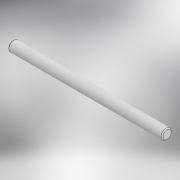
# Autodesk Inventor part: 绞杆
Saved by Autodesk Inventor 2020 (Build 240168000, 168)
## iProperties
Created: 2021-05-02
Part Number: 绞杆
Material: 常规
Document SubType Name: Modeling
Designer: Luorily
Density: 1 g/cm^3
Appearance: 默认
Author: Luorily
Autodesk Inventor part; units mm, degrees
ref_plane "YZ Plane" through (0, 0, 0) normal (1, 0, 0) x (0, 1, 0)
ref_plane "XZ Plane" through (0, 0, 0) normal (0, 1, 0) x (-1, 0, 0)
ref_plane "XY Plane" through (0, 0, 0) normal (0, 0, 1) x (1, 0, 0)
sketch "草图1" plane through (0, 0, 0) normal (0, 0, 1) x (1, 0, 0)
  line L0 (0, 0) -> (300, 0)
  line L1 (300, 0) -> (300, 10)
  line L2 (300, 10) -> (0, 10)
  line L3 (0, 10) -> (0, 0)
  dimension "d0" = 300
  dimension "d1" = 10
  constraints: 8 end point, 2 parallel, 1 horizontal, 1 perpendicular
  measures "d0" distance of L2.end L1.end
  measures "d1" distance of L1.end L0.end
revolve "旋转1" add sketch "草图1" angle 360 about axis through (0, 0, 0) along (1, 0, 0)
chamfer "倒角1" distance 2 angle 45 2 edges at (300, -10, 0) (0, -10, 0)
